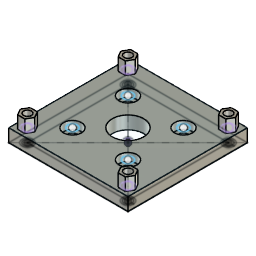
Custom C1 Bracket v3 (Autodesk Fusion 360 design; units mm, degrees)
Autodesk Fusion 360 part; units mm, degrees
note: some values were not read from the file. Set by a fixed rule: which sketch regions a step uses.
sketch "Sketch1" plane through (0, 0, 0) normal (0, 0, 1) x (1, 0, 0)
  line L0 (16, -16) -> (-16, -16)
  line L1 (-16, -16) -> (-16, 16)
  line L2 (-16, 16) -> (16, 16)
  line L3 (16, 16) -> (16, -16)
  line L4 (16, -16) -> (-16, 16) construction
  line L5 (-16, -16) -> (16, 16) construction
  circle A0 centre (-16, 16) radius 1.25
  circle A1 centre (16, 16) radius 1.25
  circle A2 centre (-16, -16) radius 1.25
  circle A3 centre (16, -16) radius 1.25
  circle A4 centre (-16, 16) radius 1.75
  circle A5 centre (16, 16) radius 1.75
  circle A6 centre (16, -16) radius 1.75
  circle A7 centre (-16, -16) radius 1.75
  line L6 (19, -19) -> (-19, -19)
  line L7 (-19, -19) -> (-19, 19)
  line L8 (-19, 19) -> (19, 19)
  line L9 (19, 19) -> (19, -19)
  line L10 (19, -19) -> (-19, 19) construction
  line L11 (-19, -19) -> (19, 19) construction
  dimension "d1" = 32
  dimension "d2" = 32
  dimension "d3" = 2.5
  dimension "d4" = 2.5
  dimension "d5" = 2.5
  dimension "d6" = 2.5
  dimension "d7" = 3.5
  dimension "d8" = 3.5
  dimension "d9" = 3.5
  dimension "d10" = 3.5
  dimension "d11" = 38
  dimension "d12" = 38
  constraint horizontal L0
  constraint perpendicular L0 L1
  constraint parallel L0 L2
  constraint parallel L1 L3
  constraint coincident L4 origin
  constraint coincident L5 origin
  constraint coincident L1.end L2.start
  constraint coincident L2.end L3.start
  constraint coincident L0.end L1.start
  constraint coincident L0.start L3.end
  constraint concentric A0 A4
  constraint concentric A1 A5
  constraint concentric A3 A6
  constraint concentric A2 A7
  constraint horizontal L6
  constraint perpendicular L6 L7
  constraint parallel L6 L8
  constraint parallel L7 L9
  constraint coincident L10 origin
  constraint coincident L11 origin
  measures "d1" distance of L1.end L2.end
  measures "d2" distance of L0.end L1.end
  measures "d3" diameter of A0
  measures "d4" diameter of A1
  measures "d5" diameter of A2
  measures "d6" diameter of A3
  measures "d7" diameter of A4
  measures "d8" diameter of A5
  measures "d9" diameter of A6
  measures "d10" diameter of A7
  measures "d11" distance of L7.end L8.end
  measures "d12" distance of L6.end L7.end
extrude "Extrude1" add sketch "Sketch1" along normal blind 4.13 contours L0 L1 L2 L3 A4 A5 A6 A7 | L6 L7 L8 L9
extrude "Extrude2" add sketch "Sketch1" along normal blind 8.13 contours L0 L1 A2 A7 | L0 L1 A2 A7 | L0 L3 A3 A6 | L0 L3 A3 A6 | L1 L2 A0 A4 | L1 L2 A0 A4 | L2 L3 A1 A5 | L2 L3 A1 A5
sketch "Sketch2" plane through (0, 0, 4.13) normal (0, 0, 1) x (-1, 0, 0)
  line L0 (-19, -19) -> (19, -19)
  line L1 (19, -19) -> (19, 19)
  line L2 (19, 19) -> (-19, 19)
  line L3 (-19, 19) -> (-19, -19)
  circle A0 centre (-16, 16) radius 1.75
  circle A1 centre (-16, -16) radius 1.75
  circle A2 centre (16, -16) radius 1.75
  circle A3 centre (16, 16) radius 1.75
  circle A4 centre (8.8388, -8.8388) radius 1.5
  circle A5 centre (-8.8388, -8.8388) radius 1.5
  circle A6 centre (8.8388, 8.8388) radius 1.5
  circle A7 centre (-8.8388, 8.8388) radius 1.5
  dimension "d32" = 3
  dimension "d33" = 3
  dimension "d34" = 3
  dimension "d35" = 3
  measures "d32" diameter of A4
  measures "d33" diameter of A5
  measures "d34" diameter of A6
  measures "d35" diameter of A7
sketch "Sketch4" plane through (0, 0, 4.13) normal (0, 0, 1) x (-1, 0, 0)
  circle A0 centre (-16, 16) radius 1.75
  circle A1 centre (-16, -16) radius 1.75
  circle A2 centre (16, -16) radius 1.75
  circle A3 centre (16, 16) radius 1.75
  line L0 (-19, -19) -> (19, -19)
  line L1 (19, -19) -> (19, 19)
  line L2 (19, 19) -> (-19, 19)
  line L3 (-19, 19) -> (-19, -19)
  line L4 (14.8453, -14) -> (13.6906, -16)
  line L5 (13.6906, -16) -> (14.8453, -18)
  line L6 (14.8453, -18) -> (17.1547, -18)
  line L7 (17.1547, -18) -> (18.3094, -16)
  line L8 (18.3094, -16) -> (17.1547, -14)
  line L9 (17.1547, -14) -> (14.8453, -14)
  line L10 (17.1547, 14) -> (18.3094, 16)
  line L11 (18.3094, 16) -> (17.1547, 18)
  line L12 (17.1547, 18) -> (14.8453, 18)
  line L13 (14.8453, 18) -> (13.6906, 16)
  line L14 (13.6906, 16) -> (14.8453, 14)
  line L15 (14.8453, 14) -> (17.1547, 14)
  line L16 (-14.8453, -18) -> (-13.6906, -16)
  line L17 (-13.6906, -16) -> (-14.8453, -14)
  line L18 (-14.8453, -14) -> (-17.1547, -14)
  line L19 (-17.1547, -14) -> (-18.3094, -16)
  line L20 (-18.3094, -16) -> (-17.1547, -18)
  line L21 (-17.1547, -18) -> (-14.8453, -18)
  line L22 (-14.8453, 14) -> (-13.6906, 16)
  line L23 (-13.6906, 16) -> (-14.8453, 18)
  line L24 (-14.8453, 18) -> (-17.1547, 18)
  line L25 (-17.1547, 18) -> (-18.3094, 16)
  line L26 (-18.3094, 16) -> (-17.1547, 14)
  line L27 (-17.1547, 14) -> (-14.8453, 14)
  point P0 (16, -16)
  point P1 (16, 16)
  point P2 (-16, -16)
  point P3 (-16, 16)
  constraint coincident P0 A2.centre
  constraint coincident P1 A3.centre
  constraint coincident A1.centre P2
  constraint coincident P3 A0.centre
extrude "Extrude5" add sketch "Sketch4" along normal blind 4 contours L4 L5 L6 L7 L8 L9 | L10 L11 L12 L13 L14 L15 | L16 L17 L18 L19 L20 L21 | L22 L23 L24 L25 L26 L27
extrude "Extrude6" cut sketch "Sketch2" against normal up to surface (4.13 mm away) contours A4 | A5 | A6 | A7
sketch "Sketch5" plane through (0, 0, 4.13) normal (0, 0, 1) x (-1, 0, 0)
  circle A0 centre (8.8388, -8.8388) radius 2.85
  circle A1 centre (-8.8388, -8.8388) radius 2.85
  circle A2 centre (-8.8388, 8.8388) radius 2.85
  circle A3 centre (8.8388, 8.8388) radius 2.85
  point P0 (8.8388, -8.8388)
  point P1 (-8.8388, -8.8388)
  point P2 (-8.8388, 8.8388)
  point P3 (8.8388, 8.8388)
  dimension "d38" = 5.7
  dimension "d39" = 5.7
  dimension "d40" = 5.7
  dimension "d41" = 5.7
  constraint coincident P0 A0.centre
  constraint coincident P1 A1.centre
  constraint coincident P2 A2.centre
  constraint coincident P3 A3.centre
  measures "d38" diameter of A0
  measures "d39" diameter of A1
  measures "d40" diameter of A2
  measures "d41" diameter of A3
extrude "Extrude7" cut sketch "Sketch5" against normal blind 2.5
sketch "Sketch6" plane through (0, 0, 4.13) normal (0, 0, 1) x (-1, 0, 0)
  circle A0 centre (0, 0) radius 5
  dimension "d44" = 10
  constraint coincident A0.centre origin
  measures "d44" diameter of A0
extrude "Extrude8" cut sketch "Sketch6" against normal up to surface (4.13 mm away)
